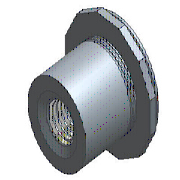
# Autodesk Inventor part: CSS-M3-4
Saved by Autodesk Inventor 2022 (Build 260153000, 153)
## iProperties
Created: 2021-02-02
Part Number: CSS-M3-4
Material: Stainless Steel
Catalog Web Link: www.pemnet.com
Description: PEM Concealed-head Standoffs CSS - Metric
Vendor: PennEngineering®
Document SubType Name: Modeling
Standard: PEM
Designer: Tomasz Krakowski
Manufacturer: PennEngineering®
Language: en-US
Size Designation: CSS-M3-4
Categories: <MemberInstance><Categories><Category DisplayName="Sheet Metal" InternalName="21944ee9-ad4d-44c9-9b1e-873eb7935d2a" Mnemonic="PEM"><Category DisplayName="Standoffs" InternalName="57b3feba-087d-4d0d-a4ac-db74cc0d8faf" Mnemonic="pemStandoffs"><CategoryParameter DisplayName="Thread Type" InternalName="4479d2df-2ba1-44f0-92d8-4a961b083ccc" Mnemonic="thrtype"/><CategoryParameter DisplayName="Hole diameter" InternalName="9f6801b2-7269-4acf-ad10-e530f6464412" Mnemonic="SMNHD"/><CategoryParameter DisplayName="Min sheet thickness" InternalName="ecb5cf93-875b-4773-8f54-c9c1078fffd0" Mnemonic="SMNMIST"/></Category></Category><Category DisplayName="DataType" InternalName="23b78d0f-2648-40c6-8793-ca6db495c9e8" Mnemonic="DATATYPE"><CategoryParameter DisplayName="DisplayName" InternalName="05415f3d-3907-474b-a020-eb9d644f4cf3" Mnemonic="DISPLAYNAME"/><CategoryParameter DisplayName="Standard" InternalName="0c0a119c-1e12-4c84-803f-101930972f5e" Mnemonic="STANDARD"/><CategoryParameter DisplayName="Description" InternalName="13903e3d-64b1-4950-80da-f627842ea37f" Mnemonic="DESCRIPTION"/><CategoryParameter DisplayName="Designation" InternalName="2675968c-4ce5-49e0-a4f5-552d29089031" Mnemonic="DESIGNATION"/><CategoryParameter DisplayName="Default Row" InternalName="2af9ec52-faaa-4026-b378-f9fa4afca842" Mnemonic="DEFAULTROW"/><CategoryParameter DisplayName="Folder Name" InternalName="3f06958e-8713-4116-9be7-ed6184ecc97b" Mnemonic="FOLDERNAME"/><CategoryParameter DisplayName="Revision Guid" InternalName="45a75005-10b1-4dfc-8d6d-dfe629f0b93c" Mnemonic="REVISIONGUID"/><CategoryParameter DisplayName="FileName" InternalName="8b46a4cc-9585-4fed-90c3-899f57e09a73" Mnemonic="FILENAME"/><CategoryParameter DisplayName="StdsOrg" InternalName="8f5914e1-4693-403f-8ab5-d37768198c9d" Mnemonic="STDSORG"/><CategoryParameter DisplayName="Family Version" InternalName="914462f6-6e19-4b14-ba84-155b9680b1d0" Mnemonic="FAMILYREVISION"/><CategoryParameter DisplayName="Standard Revision" InternalName="91d5a463-65c2-4fde-b823-3b7fea5e8e17" Mnemonic="STANDARDREVISION"/><CategoryParameter DisplayName="Member Revision" InternalName="a65d44b9-392f-4f4f-857b-e4b3d54996fe" Mnemonic="MEMBERREVISION"/><CategoryParameter DisplayName="ClipFormat" InternalName="bc51e27b-3422-4e78-93ef-cec197ddf230" Mnemonic="CLIPFORMAT"/><CategoryParameter DisplayName="Manufacturer" InternalName="cd6c7a72-a28a-4e50-99a9-2c7f4e13e5ad" Mnemonic="MANUFACTURER"/><CategoryParameter DisplayName="InternalName" InternalName="cf1d0246-76d9-4b4a-8305-fa0409afb5c1" Mnemonic="INTERNALNAME"/><CategoryParameter DisplayName="IsMetric" InternalName="e2385c5b-1ea4-4823-96a8-8de651266ec3" Mnemonic="ISMETRIC"/><Category DisplayName="Part" InternalName="c0e0b642-3bcb-4cc8-9e80-f96d35c4afa4" Mnemonic="PART"><CategoryParameter DisplayName="Part Number" InternalName="016b6077-bfbe-49bd-92c9-d8d59c39c941" Mnemonic="PARTNUMBER"/><CategoryParameter DisplayName="Stock Number" InternalName="4dba7c1c-e26c-444e-836c-b08b433409a8" Mnemonic="STOCKNUMBER"/><CategoryParameter DisplayName="Material Key" InternalName="5c9a8adb-dd2b-4535-b97f-0a94a95fe41f" Mnemonic="MATERIALKEY"/><CategoryParameter DisplayName="Material" InternalName="818a152a-d3c3-49ca-80ee-df7d91421b8e" Mnemonic="MATERIAL"/></Category></Category></Categories><FamilyTemplate Id="PEM Concealed-head Standoffs CSS - Metric"><FamilyTemplateParameters><FamilyTemplateParameter ObjectType="kUserParameterObject" ValueType="xs:double" Id="1" ObjectReferenceKey="A_"/><FamilyTemplateParameter ObjectType="kUserParameterObject" ValueType="xs:double" Id="2" ObjectReferenceKey="B"/><FamilyTemplateParameter ObjectType="kUserParameterObject" ValueType="xs:double" Id="3" ObjectReferenceKey="B_Hole"/><FamilyTemplateParameter ObjectType="kUserParameterObject" ValueType="xs:double" Id="4" ObjectReferenceKey="C_"/><FamilyTemplateParameter ObjectType="kUserParameterObject" ValueType="xs:double" Id="15" ObjectReferenceKey="H_"/><FamilyTemplateParameter ObjectType="kUserParameterObject" ValueType="xs:double" Id="16" ObjectReferenceKey="Length_Code"/><FamilyTemplateParameter ObjectType="kUserParameterObject" ValueType="xs:double" Id="17" ObjectReferenceKey="Min_Depht"/><FamilyTemplateParameter ObjectType="kUserParameterObject" ValueType="xs:double" Id="18" ObjectReferenceKey="Min_Dist"/><FamilyTemplateParameter ObjectType="kUserParameterObject" ValueType="xs:double" Id="19" ObjectReferenceKey="Min_Thick"/><FamilyTemplateParameter ObjectType="kUserParameterObject" ValueType="xs:double" Id="21" ObjectReferenceKey="Thread"/><FamilyTemplateParameter ObjectType="kUserParameterObject" ValueType="xs:double" Id="22" ObjectReferenceKey="T_"/><FamilyTemplateParameter ObjectType="kPropertyObject" ValueType="xs:string" Id="100" ObjectReferenceKey="{32853F0F-3444-11d1-9E93-0060B03C1CA6}" SubObjectId="52"/><FamilyTemplateParameter ObjectType="kPropertyObject" ValueType="xs:string" Id="105" ObjectReferenceKey="{32853F0F-3444-11d1-9E93-0060B03C1CA6}" SubObjectId="5"/><FamilyTemplateParameter ObjectType="kPartComponentDefinitionObject" ValueType="xs:string" Id="110" SubObjectId="Material"/><FamilyTemplateParameter ObjectType="kPartFeatureObject" ValueType="xs:boolean" Id="200" ObjectReferenceKey="1002000010000000d5320000000000008000000000000000" SubObjectId="Suppressed"/><FamilyTemplateParameter ObjectType="kPartFeatureObject" ValueType="xs:boolean" Id="201" ObjectReferenceKey="10020000100000007e860000000000008000000000000000" SubObjectId="Suppressed"/></FamilyTemplateParameters></FamilyTemplate><CategoryParameterMap><ParamToTemplateMap><ParamToTemplate CategoryParameter="//CategoryParameter[@InternalName='05415f3d-3907-474b-a020-eb9d644f4cf3']" ConstantValue="PEM Concealed-head Standoffs CSS - Metric"/><ParamToTemplate CategoryParameter="//CategoryParameter[@InternalName='0c0a119c-1e12-4c84-803f-101930972f5e']" ConstantValue="PEM"/><ParamToTemplate CategoryParameter="//CategoryParameter[@InternalName='13903e3d-64b1-4950-80da-f627842ea37f']" ConstantValue="PEM Concealed-head Standoffs CSS - Metric"/><ParamToTemplate CategoryParameter="//CategoryParameter[@InternalName='2af9ec52-faaa-4026-b378-f9fa4afca842']" ConstantValue="1"/><ParamToTemplate CategoryParameter="//CategoryParameter[@InternalName='3f06958e-8713-4116-9be7-ed6184ecc97b']" ConstantValue="PEM Concealed-head Standoffs CSS - Metric"/><ParamToTemplate CategoryParameter="//CategoryParameter[@InternalName='45a75005-10b1-4dfc-8d6d-dfe629f0b93c']" ConstantValue="c88120c4-173f-48fb-b06f-dfa4e7bd03eb"/><ParamToTemplate CategoryParameter="//CategoryParameter[@InternalName='8f5914e1-4693-403f-8ab5-d37768198c9d']" TemplateParameter="101"/><ParamToTemplate CategoryParameter="//CategoryParameter[@InternalName='914462f6-6e19-4b14-ba84-155b9680b1d0']" ConstantValue="11"/><ParamToTemplate CategoryParameter="//CategoryParameter[@InternalName='91d5a463-65c2-4fde-b823-3b7fea5e8e17']" TemplateParameter="103"/><ParamToTemplate CategoryParameter="//CategoryParameter[@InternalName='bc51e27b-3422-4e78-93ef-cec197ddf230']" ConstantValue="CF_INVENTOR.STDPARTS"/><ParamToTemplate CategoryParameter="//CategoryParameter[@InternalName='cd6c7a72-a28a-4e50-99a9-2c7f4e13e5ad']" ConstantValue="PennEngineering®"/><ParamToTemplate CategoryParameter="//CategoryParameter[@InternalName='cf1d0246-76d9-4b4a-8305-fa0409afb5c1']" ConstantValue="dce5beb7-6966-4528-b356-c6a25695b0b1"/><ParamToTemplate CategoryParameter="//CategoryParameter[@InternalName='e2385c5b-1ea4-4823-96a8-8de651266ec3']" ConstantValue="true"/><ParamToTemplate CategoryParameter="//CategoryParameter[@InternalName='8b46a4cc-9585-4fed-90c3-899f57e09a73']" ConstantValue="CSS-M3-4"/><ParamToTemplate CategoryParameter="//CategoryParameter[@InternalName='a65d44b9-392f-4f4f-857b-e4b3d54996fe']" ConstantValue="c4712a9b-2715-4e34-ac97-7093838b0c7f"/><ParamToTemplate CategoryParameter="//CategoryParameter[@InternalName='9f6801b2-7269-4acf-ad10-e530f6464412']" TemplateParameter="3"/><ParamToTemplate CategoryParameter="//CategoryParameter[@InternalName='2675968c-4ce5-49e0-a4f5-552d29089031']" TemplateParameter="100"/><ParamToTemplate CategoryParameter="//CategoryParameter[@InternalName='818a152a-d3c3-49ca-80ee-df7d91421b8e']" TemplateParameter="110"/><ParamToTemplate CategoryParameter="//CategoryParameter[@InternalName='ecb5cf93-875b-4773-8f54-c9c1078fffd0']" TemplateParameter="19"/><ParamToTemplate CategoryParameter="//CategoryParameter[@InternalName='016b6077-bfbe-49bd-92c9-d8d59c39c941']" TemplateParameter="105"/></ParamToTemplateMap></CategoryParameterMap></MemberInstance>
Mass: 0.485465 g
Surface Area: 1.7173 cm^2
Volume: 0.0600823 cm^3
Density: 8 g/cm^3
Appearance: Semi-Polished
IsCustomPart: 0
Author: Tomasz Krakowski
Autodesk Inventor part; units mm, degrees
ref_plane "YZ Plane" through (0, 0, 0) normal (1, 0, 0) x (0, 1, 0)
ref_plane "XZ Plane" through (0, 0, 0) normal (0, 1, 0) x (-1, 0, 0)
ref_plane "XY Plane" through (0, 0, 0) normal (0, 0, 1) x (1, 0, 0)
sketch "Sketch1" plane through (0, 0, 0) normal (1, 0, 0) x (0, 1, 0)
  line L0 (0, 0) -> (2.695, 0)
  line L1 (2.695, 0) -> (2.695, 0.1833)
  line L2 (2.695, 0.1833) -> (2.5117, 0.3667)
  line L3 (2.5117, 0.3667) -> (2.5117, 0.55)
  line L4 (2.5117, 0.55) -> (4.7625, 0.55)
  line L5 (4.7625, 0.55) -> (4.7625, 1.1)
  line L6 (4.7625, 1.1) -> (2.1, 1.1)
  line L7 (2.1, 1.1) -> (2.1, 1.2)
  arc A0 (2.1, 1.3908) -> (2.1, 1.2) centre (2.13, 1.2954) ccw
  line L8 (2.1, 1.6816) -> (2.1, 5.1)
  line L9 (2.1, 5.1) -> (0, 5.1)
  line L10 (0, 5.1) -> (0, 0)
  arc A1 (2.1, 1.6816) -> (2.1, 1.4908) centre (2.13, 1.5862) ccw
  line L11 (2.1, 1.3908) -> (2.1, 1.4908)
  dimension "d0" = 5.39
  dimension "d1" = 1.1
  dimension "d2" = 4.2
  dimension "d3" = 9.525
  dimension "d4" = 4
  dimension "d5" = 0.1
  dimension "d6" = 0.55
  dimension "d7" = 0.1833
  dimension "d8" = 0.1833
  dimension "d9" = 0.1833
  dimension "d10" = 0.03
  dimension "d11" = 0.1
  dimension "d12" = 0.1
  constraints: 24 end point, 6 parallel, 4 point on circle, 2 centre point, 2 collinear, 2 perpendicular, 1 equal radius, 1 horizontal, 1 vertical alignment
  measures "d0" diameter of L1 L10
  measures "d1" distance between parallel lines of L0 L6
  measures "d2" diameter of L7 L10
  measures "d3" diameter of L5 L10
  measures "d4" distance between parallel lines of L9 L6
  measures "d5" radius of A0
  measures "d6" distance from line of L0.end L4
  measures "d7" distance of L0.end L1.end
  measures "d8" distance of L2.end L3.end
  measures "d9" distance from line of L2.end L1
  measures "d10" distance from line of A0.centre L7
  measures "d11" distance of L6.end L7.end
  measures "d12" distance of L11.start L11.end
revolve "Revolution1" add sketch "Sketch1" angle 360 about axis through (0, 0, 5.1) along (0, 0, -1)
sketch "Sketch2" plane through (0, 0, 0.55) normal (0, 0, -1) x (-1, 0, 0)
  line L0 (0.8507, 3.175) -> (2.3243, 2.3243)
  line L1 (2.3243, 2.3243) -> (3.175, 0.8507)
  line L2 (3.175, 0.8507) -> (3.175, -0.8507)
  line L3 (3.175, -0.8507) -> (2.3243, -2.3243)
  line L4 (2.3243, -2.3243) -> (0.8507, -3.175)
  line L5 (0.8507, -3.175) -> (-0.8507, -3.175)
  line L6 (-0.8507, -3.175) -> (-2.3243, -2.3243)
  line L7 (-2.3243, -2.3243) -> (-3.175, -0.8507)
  line L8 (-3.175, -0.8507) -> (-3.175, 0.8507)
  line L9 (-3.175, 0.8507) -> (-2.3243, 2.3243)
  line L10 (-2.3243, 2.3243) -> (-0.8507, 3.175)
  line L11 (-0.8507, 3.175) -> (0.8507, 3.175)
  circle A0 centre (0, 0) radius 4.7625 projected
  dimension "d16" = 6.35
  constraints: 24 end point, 1 coincident, 1 vertical, 25 other
  measures "d16" distance between parallel lines of L2 L8
extrude "Extrusion1" cut sketch "Sketch2" against normal through all
hole "Hole1" at (0, 0, 5.1) direction (0, 0, -1) diameter 2.459 end through all countersink diameter 3.15 countersink angle 120 thread size "M3x0.5" class "6H" standard "ANSI Metric M Profile"
hole "Hole2" [suppressed]
equation "\"d0\" = C_"
equation "\"d1\" = A_"
equation "\"d2\" = B"
equation "\"d3\" = 1.5 * H_"
equation "\"d4\" = Length_Code"
equation "\"d5\" = Mark_1"
equation "\"d6\" = 0.5 * A_"
equation "\"d7\" = 0.166667 * A_"
equation "\"d8\" = 0.166667 * A_"
equation "\"d9\" = 0.166667 * A_"
equation "\"d10\" = Mark_2"
equation "\"d11\" = Mark_1"
equation "\"d12\" = Mark_1"
equation "\"d13\" = T_"
equation "\"d14\" = 1.05 * Thread"
equation "\"d53\" = Length_Code"
equation "\"d18\" = 1.05 * Thread"
equation "\"d20\" = T_"
equation "\"d16\" = H_"
equation "\"Length_Code\" = 4"
equation "\"T_\" = 4"
equation "\"A_\" = 1.1"
equation "\"B\" = 4.2"
equation "\"C_\" = 5.39"
equation "\"H_\" = 6.35"
equation "\"Mark_1\" = 0.1"
equation "\"Mark_2\" = 0.03"
equation "\"Thread\" = 3"
equation "\"Min_Thick\" = 1.6"
equation "\"B_Hole\" = 5.41"
equation "\"Min_Depht\" = 1.1"
equation "\"Min_Dist\" = 4.8"
body "Solid1"
